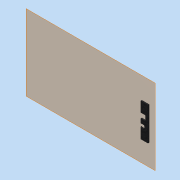
# Autodesk Inventor part: Part68
Saved by Autodesk Inventor 2017 (Build 210142000, 142)
## iProperties
Created: 2018-10-05
Part Number: Part68
Material: Generic
Document SubType Name: Modeling
Designer: mailb
Density: 1 g/cm^3
Appearance: Asphalt 2
Author: mailb
Autodesk Inventor part; units mm, degrees
ref_plane "YZ Plane" through (0, 0, 0) normal (1, 0, 0) x (0, 1, 0)
ref_plane "XZ Plane" through (0, 0, 0) normal (0, 1, 0) x (-1, 0, 0)
ref_plane "XY Plane" through (0, 0, 0) normal (0, 0, 1) x (1, 0, 0)
ref_plane "Work Plane1" through (0, 0, 0) normal (0, 0, 1) x (1, 0, 0)
sketch "Sketch1" plane through (0, 0, 0) normal (0, 0, 1) x (1, 0, 0)
  line L0 (254.7, -154.94) -> (254.7, 140.97) projected
  line L1 (291.2125, 168.0875) -> (291.2125, -168.0875) projected
  arc A0 (256.7, 31.75) -> (254.7, 29.75) centre (256.7, 29.75) ccw projected
  line L2 (254.7, 29.75) -> (254.7, 8.75) projected
  arc A1 (254.7, 8.75) -> (256.7, 6.75) centre (256.7, 8.75) ccw projected
  line L3 (256.7, 6.75) -> (276.7, 6.75) projected
  arc A2 (276.7, 6.75) -> (278.7, 8.75) centre (276.7, 8.75) ccw projected
  line L4 (278.7, 8.75) -> (278.7, 29.75) projected
  arc A3 (278.7, 29.75) -> (276.7, 31.75) centre (276.7, 29.75) ccw projected
  line L5 (276.7, 31.75) -> (256.7, 31.75) projected
  circle A4 centre (276.78, 8.75) radius 1.05 projected
  circle A5 centre (264.2, 8.75) radius 1.05 projected
  circle A6 centre (276.78, 29.75) radius 1.05 projected
  circle A7 centre (264.2, 29.75) radius 1.05 projected
  arc A8 (257.24, -13.97) -> (254.7, -16.51) centre (257.24, -16.51) ccw projected
  line L6 (254.7, -16.51) -> (254.7, -29.21) projected
  arc A9 (254.7, -29.21) -> (257.24, -31.75) centre (257.24, -29.21) ccw projected
  line L7 (257.24, -31.75) -> (269.94, -31.75) projected
  arc A10 (269.94, -31.75) -> (272.48, -29.21) centre (269.94, -29.21) ccw projected
  line L8 (272.48, -29.21) -> (272.48, -16.51) projected
  arc A11 (272.48, -16.51) -> (269.94, -13.97) centre (269.94, -16.51) ccw projected
  line L9 (269.94, -13.97) -> (257.24, -13.97) projected
  circle A12 centre (257.24, -19.05) radius 0.5 projected
  circle A13 centre (257.24, -24.13) radius 0.5 projected
  circle A14 centre (257.24, -29.21) radius 0.5 projected
  circle A15 centre (269.94, -29.21) radius 1.25 projected
  circle A16 centre (259.272, -18.923) radius 0.25 projected
  circle A17 centre (269.178, -19.304) radius 0.25 projected
  circle A18 centre (263.463, -28.702) radius 0.25 projected
  circle A19 centre (268.289, -26.67) radius 0.25 projected
  circle A20 centre (267.654, -30.861) radius 0.25 projected
  circle A21 centre (260.669, -26.797) radius 0.25 projected
  circle A22 centre (265.622, -26.035) radius 0.25 projected
  circle A23 centre (267.654, -21.717) radius 0.25 projected
  circle A24 centre (260.796, -21.971) radius 0.25 projected
  circle A25 centre (269.94, -16.51) radius 1.25 projected
  circle A26 centre (257.24, -26.67) radius 0.5 projected
  circle A27 centre (257.24, -21.59) radius 0.5 projected
  circle A28 centre (257.24, -16.51) radius 0.5 projected
  line L10 (254.7, 31.75) -> (254.7, 82.55)
  line L11 (254.7, 82.55) -> (291.2125, 82.55)
  line L12 (254.7, 31.75) -> (256.7, 31.75)
  line L13 (256.7, 6.75) -> (254.7, 6.75)
  line L14 (257.24, -13.97) -> (254.7, -13.97)
  line L15 (257.175, -31.75) -> (254.7, -31.75)
  line L16 (254.7, -31.75) -> (254.7, -82.55)
  line L17 (254.7, -82.55) -> (291.2125, -82.55)
  point P0 (0, 0)
  dimension "d0" = 50.8
  dimension "d1" = 50.8
  constraints: 16 end point, 3 horizontal, 3 point on line, 2 perpendicular, 1 tangent, 7 other
  measures "d0" distance of L10.start L10.end
  measures "d1" distance of L15.end L16.end
extrude "Extrusion1" add sketch "Sketch1" along normal blind 6.35 contours L0 L15 A9 L7 A10 L8 A11 L9 L14 L13 L3 A2 L4 A3 L5 L12 L11 L1 L17 | L0 A9 L15
body "Solid1"
